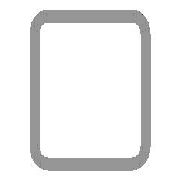
# Autodesk Inventor part: ISO 10799-2 - 80x80x3 - 3868,67
Saved by Autodesk Inventor 2025 (Build 290162010, 162A)
## iProperties
IsCustomPart: 1
Created: 2024-01-20
Part Number: ISO 10799-2 - 80x80x3 - 3868,67
Material: Steel, Mild
Description: Structural steels - Cold-formed, welded, structural hollow sections
Document SubType Name: Modeling
Standard: ISO 10799-2
Designer: pokla
Standard Revision: First edition 2011-09-15
Standards Organization: ISO
Language: en-US
Size Designation: 80x80x3
Categories: <MemberInstance><Categories><Category DisplayName="Structural Shapes" InternalName="089c4875-fa83-4c05-b084-43b9cc11f5ed" Mnemonic="GRDR"><CategoryParameter DisplayName="Mass per Length Unit" InternalName="0bb95a10-148f-4027-a459-38d7b056702a" Mnemonic="shpmass"/><CategoryParameter DisplayName="Section Area" InternalName="1ff91680-64b0-4202-b9a3-7fd3f94bba3b" Mnemonic="secarea"/><CategoryParameter DisplayName="Radius of Gyration (x)" InternalName="25778675-03e9-40c1-b6a8-4a9ed693320d" Mnemonic="gyrradx"/><CategoryParameter DisplayName="Torsional Rigidity Modulus" InternalName="26c1ec35-5026-4c63-ad0a-751cf684a536" Mnemonic="torrigmod"/><CategoryParameter DisplayName="Distance of the Center of Gravity X-X" InternalName="26c9bdb8-9c79-4b4f-a92e-8e197583c9c4" Mnemonic="grcendistX"/><CategoryParameter DisplayName="Legacy Member ID" InternalName="340afe4f-75d7-48d3-ab7d-943f3c3da468" Mnemonic="LegacyMemberID"/><CategoryParameter DisplayName="Base Length" InternalName="42e34263-8f20-4d0e-ad48-bf1385b87c24" Mnemonic="shplen"/><CategoryParameter DisplayName="Moment of Inertia (y)" InternalName="4b9f58ea-bced-460e-81ea-3d29ca5a49e3" Mnemonic="inermomy"/><CategoryParameter DisplayName="Moment of Inertia (x)" InternalName="4cd780bc-73d7-43ac-917a-579e5cbd684d" Mnemonic="inermomx"/><CategoryParameter DisplayName="Custom Base Point" InternalName="4f1d1b73-316d-484b-a3df-9cbabb16eb77" Mnemonic="shpBasePoint"/><CategoryParameter DisplayName="Shape Height" InternalName="50274e7d-5ac0-4796-92cb-c59e54983c67" Mnemonic="shpheig"/><CategoryParameter DisplayName="Section Module (y)" InternalName="59eaa5e9-d227-48dc-b6c1-6920f96e0f95" Mnemonic="secmody"/><CategoryParameter DisplayName="Section Designation" InternalName="5a64d034-428d-49c8-ba32-7619764de20f" Mnemonic="shpdes"/><CategoryParameter DisplayName="Section Module (x)" InternalName="72cfad18-cf51-4ed4-aaa7-c6b224f8419f" Mnemonic="secmodx"/><CategoryParameter DisplayName="Torsional Section Modulus" InternalName="7c55a8dc-8844-49f9-a867-cc677b30ec9a" Mnemonic="torsecmod"/><CategoryParameter DisplayName="Shape Width" InternalName="7c717d54-a18f-4666-b4d4-573cce22c62c" Mnemonic="shpwdth"/><CategoryParameter DisplayName="Second Shape Thickness" InternalName="9251a8e1-85fd-4e47-af99-afdb762317d9" Mnemonic="shpthick2"/><CategoryParameter DisplayName="FG Authored" InternalName="9c666724-f362-4ea7-ac62-f6a007de5c69" Mnemonic="shpFGAuto"/><CategoryParameter DisplayName="Distance of the Center of Gravity Y-Y" InternalName="bcc4fb17-7af4-436a-8f8c-d0aa3b0248c5" Mnemonic="grcendistY"/><CategoryParameter DisplayName="Radius of Gyration (y)" InternalName="bfa18ebe-1636-4dbe-8d42-b263e0b73184" Mnemonic="gyrrady"/><CategoryParameter DisplayName="Shape Thickness" InternalName="d109cf76-8eb4-42fc-9800-4409734adc67" Mnemonic="shpthick"/><CategoryParameter DisplayName="Coefficient of Shear Displacement" InternalName="de4c90c6-aaa8-468f-a335-6737b311b5d3" Mnemonic="shdispc"/><Category DisplayName="Square/Rectangular Tubes" InternalName="afc8e2d8-05d6-4609-8807-f98a9b7d2ed0" Mnemonic="SQRSHP"><CategoryParameter DisplayName="Section Area" InternalName="2f7f79dd-983c-4263-802a-5b6a1495fdc5" Mnemonic="secarea"/><CategoryParameter DisplayName="Section Module (x)" InternalName="50d965a6-04bf-46b9-8ace-861858d348e6" Mnemonic="secmodx"/><CategoryParameter DisplayName="Section Module (y)" InternalName="5106aeac-54a2-4159-a9af-8933dd39dba2" Mnemonic="secmody"/><CategoryParameter DisplayName="Shape Thickness" InternalName="52712fc5-f4ee-4eda-b3f2-6fce82c26419" Mnemonic="shpthick"/><CategoryParameter DisplayName="Moment of Inertia (y)" InternalName="55ec8510-8276-4c45-8f10-594e0fee7eb3" Mnemonic="inermomy"/><CategoryParameter DisplayName="Radius of Gyration (x)" InternalName="56c89926-a299-4389-a862-ac94c9691272" Mnemonic="gyrradx"/><CategoryParameter DisplayName="Radius" InternalName="5d8d062c-e28e-41c1-98da-8e5fee36da1a" Mnemonic="shprad"/><CategoryParameter DisplayName="Moment of Inertia (x)" InternalName="8c4637b6-6b69-4878-9d5d-26a32185d655" Mnemonic="inermomx"/><CategoryParameter DisplayName="Shape Width" InternalName="8c8a1782-5e80-4d77-858b-304b1c0ad1fd" Mnemonic="shpwdth"/><CategoryParameter DisplayName="Radius of Gyration (y)" InternalName="fa48a7f5-f030-40f9-a60b-de8a845b7104" Mnemonic="gyrrady"/></Category></Category><Category DisplayName="DataType" InternalName="23b78d0f-2648-40c6-8793-ca6db495c9e8" Mnemonic="DATATYPE"><CategoryParameter DisplayName="DisplayName" InternalName="05415f3d-3907-474b-a020-eb9d644f4cf3" Mnemonic="DISPLAYNAME"/><CategoryParameter DisplayName="Standard" InternalName="0c0a119c-1e12-4c84-803f-101930972f5e" Mnemonic="STANDARD"/><CategoryParameter DisplayName="Description" InternalName="13903e3d-64b1-4950-80da-f627842ea37f" Mnemonic="DESCRIPTION"/><CategoryParameter DisplayName="Designation" InternalName="2675968c-4ce5-49e0-a4f5-552d29089031" Mnemonic="DESIGNATION"/><CategoryParameter DisplayName="Default Row" InternalName="2af9ec52-faaa-4026-b378-f9fa4afca842" Mnemonic="DEFAULTROW"/><CategoryParameter DisplayName="Folder Name" InternalName="3f06958e-8713-4116-9be7-ed6184ecc97b" Mnemonic="FOLDERNAME"/><CategoryParameter DisplayName="Revision Guid" InternalName="45a75005-10b1-4dfc-8d6d-dfe629f0b93c" Mnemonic="REVISIONGUID"/><CategoryParameter DisplayName="FileName" InternalName="8b46a4cc-9585-4fed-90c3-899f57e09a73" Mnemonic="FILENAME"/><CategoryParameter DisplayName="StdsOrg" InternalName="8f5914e1-4693-403f-8ab5-d37768198c9d" Mnemonic="STDSORG"/><CategoryParameter DisplayName="Family Version" InternalName="914462f6-6e19-4b14-ba84-155b9680b1d0" Mnemonic="FAMILYREVISION"/><CategoryParameter DisplayName="Standard Revision" InternalName="91d5a463-65c2-4fde-b823-3b7fea5e8e17" Mnemonic="STANDARDREVISION"/><CategoryParameter DisplayName="Member Revision" InternalName="a65d44b9-392f-4f4f-857b-e4b3d54996fe" Mnemonic="MEMBERREVISION"/><CategoryParameter DisplayName="ClipFormat" InternalName="bc51e27b-3422-4e78-93ef-cec197ddf230" Mnemonic="CLIPFORMAT"/><CategoryParameter DisplayName="Manufacturer" InternalName="cd6c7a72-a28a-4e50-99a9-2c7f4e13e5ad" Mnemonic="MANUFACTURER"/><CategoryParameter DisplayName="InternalName" InternalName="cf1d0246-76d9-4b4a-8305-fa0409afb5c1" Mnemonic="INTERNALNAME"/><CategoryParameter DisplayName="IsMetric" InternalName="e2385c5b-1ea4-4823-96a8-8de651266ec3" Mnemonic="ISMETRIC"/><Category DisplayName="Part" InternalName="c0e0b642-3bcb-4cc8-9e80-f96d35c4afa4" Mnemonic="PART"><CategoryParameter DisplayName="Part Number" InternalName="016b6077-bfbe-49bd-92c9-d8d59c39c941" Mnemonic="PARTNUMBER"/><CategoryParameter DisplayName="Stock Number" InternalName="4dba7c1c-e26c-444e-836c-b08b433409a8" Mnemonic="STOCKNUMBER"/><CategoryParameter DisplayName="Material Key" InternalName="5c9a8adb-dd2b-4535-b97f-0a94a95fe41f" Mnemonic="MATERIALKEY"/><CategoryParameter DisplayName="Material" InternalName="818a152a-d3c3-49ca-80ee-df7d91421b8e" Mnemonic="MATERIAL"/></Category></Category><Category DisplayName="LegacyMap" InternalName="cd87c42b-3e48-431e-b5c0-1cbeb14dfe77" Mnemonic="LEGACYMAP"><CategoryParameter DisplayName="unique DA member ID" InternalName="0918ad47-427f-4fed-ae26-24c81c58f590" Mnemonic="DACOOKIE"/><CategoryParameter DisplayName="Merge11 ID" InternalName="0ee8fb18-e2ed-4f39-96f6-1f4b5f50aa71" Mnemonic="MERGE11"/><CategoryParameter DisplayName="unique CC member ID" InternalName="5193edd4-b2b0-4ab4-9d54-de900eee34e0" Mnemonic="CCCOOKIE"/><CategoryParameter DisplayName="Split ID" InternalName="72b5c83c-be7f-45c4-ae51-9160ea6deb26" Mnemonic="SPLIT"/><CategoryParameter DisplayName="MemberID" InternalName="8e5e0294-fc51-4c8f-b3d7-003dc5ed94f6" Mnemonic="MEMBERID"/><CategoryParameter DisplayName="CatalogName" InternalName="d99d1e27-aa94-4de2-af4c-c348882a6f4f" Mnemonic="CATALOGNAME"/><CategoryParameter DisplayName="FamilyNumber" InternalName="e705e1f4-09cb-413e-91f9-551b4188271e" Mnemonic="FAMILYNUMBER"/></Category></Categories><FamilyTemplate Id="gp0602"><FamilyTemplateParameters><FamilyTemplateParameter ObjectType="kUserParameterObject" ValueType="xs:double" Id="1" ObjectReferenceKey="G_H"/><FamilyTemplateParameter ObjectType="kUserParameterObject" ValueType="xs:double" Id="2" ObjectReferenceKey="B_L"/><FamilyTemplateParameter ObjectType="kUserParameterObject" ValueType="xs:double" Id="7" ObjectReferenceKey="G_W"/><FamilyTemplateParameter ObjectType="kUserParameterObject" ValueType="xs:double" Id="8" ObjectReferenceKey="G_T"/><FamilyTemplateParameter ObjectType="kUserParameterObject" ValueType="xs:double" Id="9" ObjectReferenceKey="G_IR"/><FamilyTemplateParameter ObjectType="kUserParameterObject" ValueType="xs:double" Id="117" ObjectReferenceKey="MAS"/><FamilyTemplateParameter ObjectType="kPropertyObject" ValueType="xs:string" Id="100" ObjectReferenceKey="{32853F0F-3444-11d1-9E93-0060B03C1CA6}" SubObjectId="52"/><FamilyTemplateParameter ObjectType="kPropertyObject" ValueType="xs:string" Id="105" ObjectReferenceKey="{32853F0F-3444-11d1-9E93-0060B03C1CA6}" SubObjectId="5"/><FamilyTemplateParameter ObjectType="kPartComponentDefinitionObject" ValueType="xs:string" Id="110" SubObjectId="Material"/><FamilyTemplateParameter ObjectType="kPropertyObject" ValueType="xs:string" Id="112" ObjectReferenceKey="{32853F0F-3444-11d1-9E93-0060B03C1CA6}" SubObjectId="55"/></FamilyTemplateParameters></FamilyTemplate><CategoryParameterMap><ParamToTemplateMap><ParamToTemplate CategoryParameter="//CategoryParameter[@InternalName='05415f3d-3907-474b-a020-eb9d644f4cf3']" ConstantValue="ISO 10799-2 (Square)"/><ParamToTemplate CategoryParameter="//CategoryParameter[@InternalName='cf1d0246-76d9-4b4a-8305-fa0409afb5c1']" ConstantValue="B3306885-1DD1-481B-BD24-E3DFD0254DB6"/><ParamToTemplate CategoryParameter="//CategoryParameter[@InternalName='3f06958e-8713-4116-9be7-ed6184ecc97b']" ConstantValue="ISO 10799-2(S)"/><ParamToTemplate CategoryParameter="//CategoryParameter[@InternalName='914462f6-6e19-4b14-ba84-155b9680b1d0']" ConstantValue="10"/><ParamToTemplate CategoryParameter="//CategoryParameter[@InternalName='bc51e27b-3422-4e78-93ef-cec197ddf230']" ConstantValue="CF_INVENTOR.STDPARTS"/><ParamToTemplate CategoryParameter="//CategoryParameter[@InternalName='e2385c5b-1ea4-4823-96a8-8de651266ec3']" ConstantValue="true"/><ParamToTemplate CategoryParameter="//CategoryParameter[@InternalName='13903e3d-64b1-4950-80da-f627842ea37f']" ConstantValue="Structural steels - Cold-formed, welded, structural hollow sections"/><ParamToTemplate CategoryParameter="//CategoryParameter[@InternalName='8f5914e1-4693-403f-8ab5-d37768198c9d']" ConstantValue="ISO"/><ParamToTemplate CategoryParameter="//CategoryParameter[@InternalName='0c0a119c-1e12-4c84-803f-101930972f5e']" ConstantValue="ISO 10799-2"/><ParamToTemplate CategoryParameter="//CategoryParameter[@InternalName='cd6c7a72-a28a-4e50-99a9-2c7f4e13e5ad']" TemplateParameter="104"/><ParamToTemplate CategoryParameter="//CategoryParameter[@InternalName='91d5a463-65c2-4fde-b823-3b7fea5e8e17']" ConstantValue="First edition 2011-09-15"/><ParamToTemplate CategoryParameter="//CategoryParameter[@InternalName='45a75005-10b1-4dfc-8d6d-dfe629f0b93c']" ConstantValue="0248128b-30b5-4ec4-8b02-06538bffa172"/><ParamToTemplate CategoryParameter="//CategoryParameter[@InternalName='2af9ec52-faaa-4026-b378-f9fa4afca842']" ConstantValue="1"/><ParamToTemplate CategoryParameter="//CategoryParameter[@InternalName='9c666724-f362-4ea7-ac62-f6a007de5c69']" ConstantValue="1"/><ParamToTemplate CategoryParameter="//CategoryParameter[@InternalName='8b46a4cc-9585-4fed-90c3-899f57e09a73']" ConstantValue="ISO 10799-2 - 80x80x3 - 0,001"/><ParamToTemplate CategoryParameter="//CategoryParameter[@InternalName='a65d44b9-392f-4f4f-857b-e4b3d54996fe']" ConstantValue="8883686C-8815-48C6-B75A-74A96244C854"/><ParamToTemplate CategoryParameter="//CategoryParameter[@InternalName='8c4637b6-6b69-4878-9d5d-26a32185d655']" ConstantValue="87,8"/><ParamToTemplate CategoryParameter="//CategoryParameter[@InternalName='56c89926-a299-4389-a862-ac94c9691272']" ConstantValue="3,12"/><ParamToTemplate CategoryParameter="//CategoryParameter[@InternalName='50d965a6-04bf-46b9-8ace-861858d348e6']" ConstantValue="22,0"/><ParamToTemplate CategoryParameter="//CategoryParameter[@InternalName='2f7f79dd-983c-4263-802a-5b6a1495fdc5']" ConstantValue="9,01"/><ParamToTemplate CategoryParameter="//CategoryParameter[@InternalName='7c55a8dc-8844-49f9-a867-cc677b30ec9a']" ConstantValue="33,0"/><ParamToTemplate CategoryParameter="//CategoryParameter[@InternalName='26c1ec35-5026-4c63-ad0a-751cf684a536']" ConstantValue="140"/><ParamToTemplate CategoryParameter="//CategoryParameter[@InternalName='de4c90c6-aaa8-468f-a335-6737b311b5d3']" ConstantValue="2,2807563"/><ParamToTemplate CategoryParameter="//CategoryParameter[@InternalName='5a64d034-428d-49c8-ba32-7619764de20f']" ConstantValue="80x80x3"/><ParamToTemplate CategoryParameter="//CategoryParameter[@InternalName='8e5e0294-fc51-4c8f-b3d7-003dc5ed94f6']" ConstantValue="30"/><ParamToTemplate CategoryParameter="//CategoryParameter[@InternalName='72b5c83c-be7f-45c4-ae51-9160ea6deb26']" ConstantValue="3626dfda-4397-4799-877a-2fe52dc968f5"/><ParamToTemplate CategoryParameter="//CategoryParameter[@InternalName='42e34263-8f20-4d0e-ad48-bf1385b87c24']" TemplateParameter="2"/><ParamToTemplate CategoryParameter="//CategoryParameter[@InternalName='2675968c-4ce5-49e0-a4f5-552d29089031']" TemplateParameter="100"/><ParamToTemplate CategoryParameter="//CategoryParameter[@InternalName='50274e7d-5ac0-4796-92cb-c59e54983c67']" TemplateParameter="1"/><ParamToTemplate CategoryParameter="//CategoryParameter[@InternalName='818a152a-d3c3-49ca-80ee-df7d91421b8e']" TemplateParameter="110"/><ParamToTemplate CategoryParameter="//CategoryParameter[@InternalName='016b6077-bfbe-49bd-92c9-d8d59c39c941']" TemplateParameter="105"/><ParamToTemplate CategoryParameter="//CategoryParameter[@InternalName='4dba7c1c-e26c-444e-836c-b08b433409a8']" TemplateParameter="112"/></ParamToTemplateMap></CategoryParameterMap></MemberInstance>
Stock Number: 80x80x3
Density: 7.85 g/cm^3
Appearance: Default
_CCFamilyMember: 30
_CCFamilyDisplayName: ISO 10799-2 (Square) - Structural steels - Cold-formed, welded, structural hollow sections
_FrameMemberDoc: Frame Member File
_Version: 15.0.0
_GetPNFromCC: 1
G_L: 3868,673 mm
G_W: 80,000 mm
G_H: 80,000 mm
Author: pokla
Autodesk Inventor part; units mm, degrees
note: some values were not read from the file. Left out: dimensions or parameters whose unit could not be read.
ref_plane "YZ Plane" through (0, 0, 0) normal (1, 0, 0) x (0, 1, 0)
ref_plane "Start Plane" through (0, 0, 0) normal (0, 0, 1) x (1, 0, 0)
ref_plane "End Plane" through (0, 0, 3868.6729) normal (0, 0, 1) x (1, 0, 0)
sketch "Sketch" plane through (0, 0, 0) normal (0, 0, 1) x (1, 0, 0)
  line L0 (-40, -34) -> (-40, 34)
  line L1 (-34, 40) -> (34, 40)
  line L2 (40, 34) -> (40, -34)
  line L3 (34, -40) -> (-34, -40)
  arc A0 (-40, -34) -> (-34, -40) centre (-34, -34) ccw
  arc A1 (40, 34) -> (34, 40) centre (34, 34) ccw
  arc A2 (-34, 40) -> (-40, 34) centre (-34, 34) ccw
  arc A3 (34, -40) -> (40, -34) centre (34, -34) ccw
  arc A4 (-34, 37) -> (-37, 34) centre (-34, 34) ccw
  line L4 (-34, 37) -> (34, 37)
  arc A5 (37, 34) -> (34, 37) centre (34, 34) ccw
  line L5 (37, 34) -> (37, -34)
  arc A6 (34, -37) -> (37, -34) centre (34, -34) ccw
  line L6 (34, -37) -> (-34, -37)
  arc A7 (-37, -34) -> (-34, -37) centre (-34, -34) ccw
  line L7 (-37, -34) -> (-37, 34)
  line L8 (0, 57.7397) -> (0, -57.7397) construction
  line L9 (-57.7397, 0) -> (57.7397, 0) construction
  dimension "d7" = 6
  dimension "d9" = 80
  dimension "d11" = 80
  dimension "d12" = 3
  dimension "d15" = 40
  dimension "d16" = 40
  constraints: 16 end point, 16 point on circle, 8 centre point, 8 tangent, 4 parallel, 3 equal radius, 2 perpendicular, 7 other
  measures "d7" radius of A0
  measures "d9" distance between parallel lines of L0 L2
  measures "d11" distance between parallel lines of L1 L3
  measures "d12" distance between parallel lines of L2 L5
  measures "d15" distance between parallel lines of L8 L2
  measures "d16" distance between parallel lines of L1 L9
extrude "Body" add sketch "Sketch" along normal up to surface (3868.6729 mm away) from surface at 0
sketch "Sketch3" plane through (0, 0, 0) normal (0, 0, 1) x (1, 0, 0)
  line L0 (0, 0) -> (10, 0)
ref_plane "Work Plane3" through (0, 0, 0) normal (0, -1, 0) x (1, 0, 0)
sketch "Sketch4" plane through (0, 0, 0) normal (0, -1, 0) x (1, 0, 0)
  line L0 (-2, 0) -> (12, 0) projected
  line L1 (-2, 3868.6729) -> (12, 3868.6729) projected
  dimension "d18" = 3868.673
  measures "d18" distance between parallel lines of L0 L1
equation "\"d7\" = G_IR"
equation "\"d9\" = G_W"
equation "\"d11\" = G_H"
equation "\"d12\" = G_T"
equation "\"d15\" = 0.5 * d9"
equation "\"d16\" = 0.5 * d11"
equation "\"d3\" = G_L"
equation "\"G_W\" = 80"
equation "\"G_H\" = 80"
equation "\"G_T\" = 3"
equation "\"G_IR\" = 6"
equation "\"G_L\" = d18"
equation "\"G_OFFSET_START\" = 0"
equation "\"G_OFFSET_END\" = 0"
equation "\"d14\" = G_OFFSET_END + B_L"
equation "\"B_L\" = 3868.67295"
body "Solid1"
